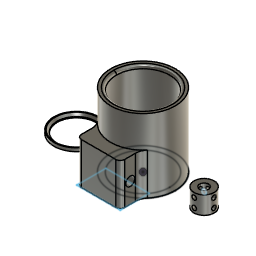
ping_pong_pvc_attatchment v2 (Autodesk Fusion 360 design; units mm, degrees)
Autodesk Fusion 360 part; units mm, degrees
note: some values were not read from the file. Set by a fixed rule: which sketch regions a step uses.
sketch "Sketch1" plane through (0, 0, 0) normal (0, 0, 1) x (1, 0, 0)
  circle A0 centre (0, 0) radius 29
  circle A1 centre (0, 0) radius 24
  line L0 (-19.525, -13.9562) -> (19.525, -13.9562)
  line L1 (19.525, -13.9562) -> (19.525, -40)
  line L2 (19.525, -40) -> (-19.525, -40)
  line L3 (-19.525, -40) -> (-19.525, -13.9562)
  dimension "d1" = 58
  dimension "d2" = -5
  constraint coincident A0.centre A1.centre
  constraint horizontal L0
  constraint vertical L1
  constraint horizontal L2
  constraint vertical L3
  constraint coincident A1 L0.start
  constraint coincident A1 L0.end
  measures "d1" diameter of A0
sketch "Sketch2" plane through (0, 0, 0) normal (1, 0, 0) x (0, 1, 0)
  circle A0 centre (-31, 18) radius 4.075
  dimension "d3" = 8.15
  measures "d3" diameter of A0
extrude "Extrude1" add sketch "Sketch1" along normal blind 37.5 contours A0 A1 L1 L3 | A0 A1 L1 L3 | A0 L1 L2 L3 makes body 1
extrude "Extrude2" cut sketch "Sketch2" along normal mid plane 50 bodies 1
extrude "Extrude3" add sketch "Sketch1" along normal blind 18.5 from surface at 37.5 contours A0 A1 L1 L3 | A0 A1 L1 L3 bodies 1
sketch "Sketch3" plane through (0, 0, 0) normal (0, 0, 1) x (1, 0, 0)
extrude "Extrude4" add 1 faces at (2.0071, -27.2067, 56) along direction (0, 0, 1) blind 10 on bodies 1 bodies 1
sketch "Sketch4" plane through (0, 0, 0) normal (0, 0, 1) x (1, 0, 0)
  circle A0 centre (-60, 0) radius 20.1
  circle A1 centre (-60, 0) radius 17.2627
  dimension "d13" = 40.2
  constraint concentric A0 A1
  measures "d13" diameter of A0
extrude "Extrude5" add sketch "Sketch4" along normal blind 3 separate body makes body 2
chamfer "Chamfer1" distance 2 angle 45 1 edges at (-76.0945, 6.2425, 3) on bodies 2
fillet "Fillet1" radius 12.5 2 edges at (-19.525, -21.4424, 18.75) (19.525, -21.4424, 18.75) on bodies 1
fillet "Fillet2" radius 2.5 tangency weight 1.39052 1 edges at (-22.3759, 8.6788, 66) on bodies 1
fillet "Fillet3" radius 4 2 edges at (19.525, -40, 18.75) (-19.525, -40, 18.75) on bodies 1
sketch "Sketch5" plane through (0, 0, 0) normal (0, 0, 1) x (1, 0, 0)
  circle A0 centre (55, 0) radius 4.05
  circle A1 centre (55, 0) radius 9.05
  dimension "d23" = 8.1
  dimension "d24" = 5
  measures "d23" diameter of A0
extrude "Extrude6" add sketch "Sketch5" along normal blind 16 separate body makes body 3
sketch "Sketch6" plane through (0, 0, 0) normal (0, 1, 0) x (1, 0, 0)
  circle A0 centre (55, -12) radius 2
  dimension "d27" = 4
  measures "d27" diameter of A0
extrude "Extrude7" cut sketch "Sketch6" along normal mid plane 24 bodies 3
pattern_circular "C-Pattern1" count 4 over 360 about axis through (55, 0, 0) along (0, 0, 1) of "Extrude7"
pattern_linear "R-Pattern1" count 1 spacing 0 along (1, 0, 0) count 2 spacing 8 along (0, 0, -1) of "Extrude7", "C-Pattern1"
